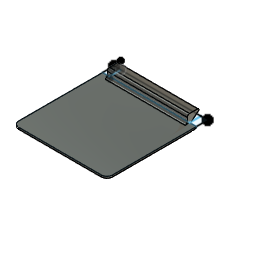
ElectronicDrawer_Divider_Middle v3 (Autodesk Fusion 360 design; units mm, degrees)
Autodesk Fusion 360 part; units mm, degrees
note: some values were not read from the file. Chosen so that the rebuilt part matches the saved one: which face or edge a step refers to. Set by a fixed rule: which sketch regions a step uses.
sketch "Sketch1" plane through (0, 0, 0) normal (0, 0, 1) x (1, 0, 0)
  line L0 (0, 0) -> (82.7, 0)
  line L1 (82.7, 0) -> (82.7, -89)
  line L2 (82.7, -89) -> (0, -89)
  line L3 (0, -89) -> (0, 0)
  line L4 (76.7, -10) -> (76.7, -74.5)
  line L5 (6, -74.5) -> (6, -10)
  line L6 (6, -10) -> (76.7, -10)
  line L7 (76.7, -74.5) -> (6, -74.5)
  dimension "d1" = 82.7
  dimension "d2" = 89
  constraint horizontal L0
  constraint vertical L1
  constraint horizontal L2
  constraint vertical L3
  constraint coincident L0.start L3.end
  measures "d1" distance of L0.start L0.end
  measures "d2" distance of L0.start L2.end
extrude "Extrude1" add sketch "Sketch1" along normal blind 1.5 makes body 1
extrude "Extrude2" add sketch "Sketch1" along normal up to surface (1.5 mm away) contours L4 L5 L6 L7 bodies 1
fillet "Fillet1" radius 5 2 edges at (82.7, -89, 0.75) (0, -89, 0.75) on bodies 1
fillet "Fillet2" [no effect]
sketch "Sketch2" plane through (0, 0, 1.5) normal (0, 0, 1) x (-1, 0, 0)
  arc A0 (0, 84) -> (-5, 89) centre (-5, 84) ccw
  line L0 (-5, 89) -> (-77.7, 89)
  arc A1 (-77.7, 89) -> (-82.7, 84) centre (-77.7, 84) ccw
  line L1 (-82.7, 84) -> (-82.7, 0)
  line L2 (-82.7, 0) -> (0, 0)
  line L3 (0, 0) -> (0, 84)
  line L4 (-6, 0) -> (-76.7, 0)
  line L5 (-76.7, 0) -> (-76.7, 10)
  line L6 (-76.7, 10) -> (-6, 10)
  line L7 (-6, 10) -> (-6, 0)
  line L8 (-76.7, 10) -> (-82.7, 10)
  line L9 (-82.7, 10) -> (-82.7, 0)
  line L10 (-82.7, 0) -> (-76.7, 0)
  line L11 (-76.7, 0) -> (-76.7, 10)
  line L12 (-6, 10) -> (0, 10)
  line L13 (0, 10) -> (0, 0)
  line L14 (0, 0) -> (-6, 0)
  line L15 (-6, 0) -> (-6, 10)
  constraint horizontal L4
  constraint vertical L5
  constraint horizontal L6
  constraint vertical L7
  constraint coincident L2 L4.start
  constraint horizontal L8
  constraint vertical L9
  constraint horizontal L10
  constraint vertical L11
  constraint coincident L1.end L2.start
  constraint horizontal L12
  constraint vertical L13
  constraint horizontal L14
  constraint vertical L15
  constraint coincident L2.end L3.start
extrude "Extrude3" cut sketch "Sketch2" against normal blind 6 contours L2 L3 L7 L12 L13 L14 L15 bodies 1
extrude "Extrude4" cut sketch "Sketch2" against normal blind 10 contours L1 L2 L5 L8 L9 L10 L11 bodies 1
extrude "Extrude5" add sketch "Sketch2" along normal blind 7 contours L2 L4 L5 L6 L7 L11 L15 bodies 1
sketch "Sketch3" plane through (6, 0, 0) normal (-1, 0, 0) x (0, -1, 0)
  line L0 (0, 0) -> (10, 0)
  line L1 (10, 0) -> (10, 1.5)
  line L2 (10, 1.5) -> (10, 8.5)
  line L3 (10, 8.5) -> (0, 8.5)
  line L4 (0, 8.5) -> (0, 0)
  line L5 (10, 0) -> (0, 8.5)
  constraint coincident L0.end L1.start
  constraint coincident L3.end L4.start
ref_plane "WorkPlane1" through (6, 0, 8.5) normal (0, 0.647648, -0.761939) x (-1, 0, 0)
split "Split1" by plane through (6, 0, 8.5) normal (0, 0.647648, -0.761939) bodies 1 makes body 2 at (53.1333, -6.6667, 0)
extrude "Extrude6" add 1 faces at (53.1333, -10, 3.8333) along direction (0, -1, 0) blind 2 on bodies 1 bodies 1
fillet "Fillet3" radius 8.5 1 edges at (41.35, -10, 0) on bodies 1
fillet "Fillet4" radius 1 1 edges at (41.35, 0, 8.5) on bodies 1
fillet "Fillet5" [no effect]
fillet "Fillet6" radius 2 2 edges at (41.35, -12, 1.5) (41.35, -12, 8.5) on bodies 1
hidden bodies 2
